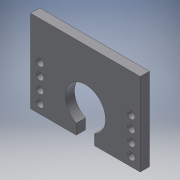
# Autodesk Inventor part: Extruder bracket
Saved by Autodesk Inventor 2019 (Build 230136000, 136)
## iProperties
Created: 2018-10-20
Part Number: Extruder bracket
Material: Generic
Document SubType Name: Modeling
Designer: LillaHunden
Density: 1 g/cm^3
Appearance: Default
Author: LillaHunden
Autodesk Inventor part; units mm, degrees
ref_plane "YZ Plane" through (0, 0, 0) normal (1, 0, 0) x (0, 1, 0)
ref_plane "XZ Plane" through (0, 0, 0) normal (0, 1, 0) x (-1, 0, 0)
ref_plane "XY Plane" through (0, 0, 0) normal (0, 0, 1) x (1, 0, 0)
sketch "Sketch1" plane through (0, 0, 0) normal (0, 0, 1) x (1, 0, 0)
  circle A0 centre (0, 0) radius 11.0071 projected
  circle A1 centre (25.0416, -10.5) radius 2 projected
  circle A2 centre (25.0416, -4) radius 2 projected
  circle A3 centre (25.0416, 2.5) radius 2 projected
  circle A4 centre (25.0416, 9) radius 2 projected
  circle A5 centre (-24.9584, 9) radius 2 projected
  circle A6 centre (-24.9584, 2.5) radius 2 projected
  circle A7 centre (-24.9584, -4) radius 2 projected
  circle A8 centre (-24.9584, -10.5) radius 2 projected
  arc A9 (-26, 15.5) -> (-30, 11.5) centre (-26, 11.5) ccw projected
  line L0 (-30, 11.5) -> (-30, -11.5) projected
  arc A10 (-30, -11.5) -> (-26, -15.5) centre (-26, -11.5) ccw projected
  line L1 (-26, -15.5) -> (26, -15.5) projected
  arc A11 (26, -15.5) -> (30, -11.5) centre (26, -11.5) ccw projected
  line L2 (30, -11.5) -> (30, 11.5) projected
  arc A12 (30, 11.5) -> (26, 15.5) centre (26, 11.5) ccw projected
  line L3 (26, 15.5) -> (-26, 15.5) projected
  line L4 (30, -15.5) -> (-30, -15.5)
  line L5 (-30, -15.5) -> (-30, 29.8174)
  line L6 (-30, 29.8174) -> (30, 29.8174)
  line L7 (30, 29.8174) -> (30, -15.5)
  point P0 (0, 0)
  dimension "d0" = 60
  constraints: 8 end point, 2 parallel, 1 horizontal, 1 perpendicular, 1 point on line
  measures "d0" distance of L5.end L6.end
extrude "Extrusion1" add sketch "Sketch1" along normal blind 5
sketch "Sketch2" plane through (0, 0, 5) normal (0, 0, 1) x (1, 0, 0)
  line L0 (-30, -15.5) -> (30, -15.5) projected
  line L1 (5, -15.5) -> (-5, -15.5)
  line L2 (-5, -15.5) -> (-5, -8.3243)
  line L3 (-5, -8.3243) -> (5, -8.3243)
  line L4 (5, -8.3243) -> (5, -15.5)
  line L5 (0, 0) -> (0, -2.4167)
  dimension "d4" = 10
  constraints: 10 end point, 2 parallel, 1 horizontal, 1 perpendicular, 1 point on line, 1 vertical, 1 other
  measures "d4" distance of L2.end L3.end
extrude "Extrusion2" cut sketch "Sketch2" against normal through all
body "Solid1"
